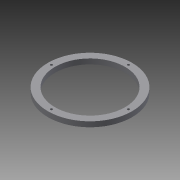
# Autodesk Inventor part: open3
Saved by Autodesk Inventor 2015 (Build 190159000, 159)
## iProperties
Created: 2015-02-17
Part Number: open3
Material: Generic
Document SubType Name: Modeling
Designer: Hanjie
Density: 1 g/cm^3
Appearance: Default
Author: Hanjie
Autodesk Inventor part; units mm, degrees
ref_plane "YZ Plane" through (0, 0, 0) normal (1, 0, 0) x (0, 1, 0)
ref_plane "XZ Plane" through (0, 0, 0) normal (0, 1, 0) x (-1, 0, 0)
ref_plane "XY Plane" through (0, 0, 0) normal (0, 0, 1) x (1, 0, 0)
sketch "Sketch1" plane through (0, 0, 0) normal (0, 1, 0) x (-1, 0, 0)
  circle A0 centre (0, 0) radius 45.72
  dimension "d0" = 91.44
  constraints: 1 centre point, 1 coincident
  measures "d0" diameter of A0
extrude "Extrusion1" add sketch "Sketch1" along normal blind 5.588
sketch "Sketch2" plane through (0, 5.588, 0) normal (0, 1, 0) x (1, 0, 0)
  circle A0 centre (0, 0) radius 38.1
  line L0 (0, 0) -> (-41.91, 0)
  line L1 (0, 0) -> (0, 41.91)
  line L2 (0, 0) -> (41.91, 0)
  line L3 (0, 0) -> (0, -41.91)
  circle A1 centre (-41.91, 0) radius 1.27
  circle A2 centre (0, 41.91) radius 1.27
  circle A3 centre (41.91, 0) radius 1.27
  circle A4 centre (0, -41.91) radius 1.27
  dimension "d3" = 76.2
  dimension "d4" = 41.91
  dimension "d5" = 41.91
  dimension "d6" = 41.91
  dimension "d7" = 41.91
  dimension "d8" = 2.54
  dimension "d9" = 2.54
  dimension "d10" = 2.54
  dimension "d11" = 2.54
  constraints: 8 end point, 5 centre point, 5 coincident, 2 vertical, 1 horizontal, 1 perpendicular
  measures "d3" diameter of A0
  measures "d4" distance of L0.start L0.end
  measures "d5" distance of L0.start L1.end
  measures "d6" distance of L0.start L2.end
  measures "d7" distance of L0.start L3.end
  measures "d8" diameter of A1
  measures "d9" diameter of A2
  measures "d10" diameter of A3
  measures "d11" diameter of A4
extrude "Extrusion2" cut sketch "Sketch2" against normal blind 5.588
body "Solid1"
